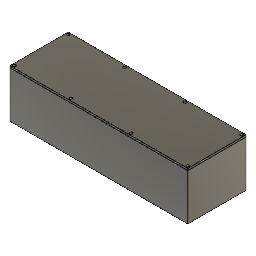
piPlayer (Autodesk Fusion 360 design; units mm, degrees)
Autodesk Fusion 360 part; units mm, degrees
note: some values were not read from the file. Set by a fixed rule: which sketch regions a step uses.
sketch "Sketch1" plane through (0, 0, 0) normal (0, 0, 1) x (1, 0, 0) in component "Box"
  line L0 (0, 26.5) -> (-38, 26.5)
  line L1 (-38, 26.5) -> (-38, -26.5)
  line L2 (-38, -26.5) -> (0, -26.5)
  line L3 (0, -26.5) -> (0, 26.5)
  line L4 (-38, -26.5) -> (-91, -26.5)
  line L5 (-91, -26.5) -> (-91, 26.5)
  line L6 (-91, 26.5) -> (-38, 26.5)
  line L7 (-91, 26.5) -> (-38, -26.5) construction
  line L8 (-38, 26.5) -> (-91, -26.5) construction
  circle A0 centre (-64.5, 0) radius 26.5
  circle A1 centre (-85.7132, 21.2132) radius 2
  circle A2 centre (-43.2868, 21.2132) radius 2
  circle A3 centre (-43.2868, -21.2132) radius 2
  circle A4 centre (-85.7132, -21.2132) radius 2
  line L9 (0, 31.5) -> (-96, 31.5)
  line L10 (-96, 31.5) -> (-96, -31.5)
  line L11 (-96, -31.5) -> (0, -31.5)
  line L12 (0, -31.5) -> (0, -26.5)
  line L13 (0, 31.5) -> (0, 26.5)
  line L14 (-36, -26.5) -> (-36, 26.5)
  circle A5 centre (-29, 0.4958) radius 4
  circle A6 centre (-29, 0.4958) radius 3
  circle A7 centre (-28.5622, -22.5) radius 1.5
  circle A8 centre (-28.5622, -22.5) radius 4
  dimension "d10" = 38
  dimension "d11" = 53
  dimension "d12" = 53
  dimension "d13" = 53
  dimension "d14" = 4
  dimension "d15" = 60
  dimension "d16" = 5
  dimension "d17" = 5
  dimension "d18" = 5
  dimension "d23" = 2
  dimension "d30" = 8
  dimension "d31" = 6
  dimension "d32" = 29
  dimension "d53" = 23
  dimension "d54" = 3
  dimension "d55" = 8
  constraint horizontal L0
  constraint vertical L1
  constraint horizontal L2
  constraint vertical L3
  constraint coincident origin L3
  constraint horizontal L4
  constraint vertical L5
  constraint horizontal L6
  constraint collinear L0 L6
  constraint midpoint L8 A0.centre
  constraint midpoint origin L3
  constraint coincident L7 A1.centre
  constraint coincident L8 A2.centre
  constraint coincident L7 A3.centre
  constraint coincident L8 A4.centre
  constraint equal A1 A2
  constraint equal A1 A3
  constraint equal A1 A4
  constraint horizontal A1.centre A2.centre
  constraint vertical A2.centre A3.centre
  constraint horizontal A3.centre A4.centre
  constraint perpendicular L3 L9
  constraint perpendicular L9 L10
  constraint perpendicular L3 L11
  constraint perpendicular L2 L12
  constraint perpendicular L0 L13
  constraint coincident L2 L14.start
  constraint coincident L0 L14.end
  constraint perpendicular L0 L14
  constraint concentric A5 A6
  constraint concentric A7 A8
  constraint tangent L2 A8
  measures "d10" distance of L0.start L0.end
  measures "d11" distance of L5.end L0.end
  measures "d12" distance of L4.end L5.end
  measures "d13" diameter of A0
  measures "d14" diameter of A1
  measures "d15" distance of A2.centre A4.centre
  measures "d16" distance of L0 L9
  measures "d17" distance of L5 L10
  measures "d18" distance of L4 L11
  measures "d23" distance of L1 L14
  measures "d30" diameter of A5
  measures "d31" diameter of A6
  measures "d32" distance of L3 A5.centre
  measures "d53" distance of A5.centre A7.centre
  measures "d54" diameter of A7
  measures "d55" diameter of A8
extrude "Extrude1" add sketch "Sketch1" along normal blind 2 contours A8 | L0 L2 L3 L14 | L0 L1 L2 L14 | L1 L6 A0 | L1 L4 A0 | L5 L6 A0 | L4 L5 A0 | A5 | A6 | A7 makes body 1 at (-12.6914, -0.6601, 0) in component "Box"
extrude "Extrude2" add sketch "Sketch1" along normal blind 50 contours L0 L2 L4 L5 L6 L9 L10 L11 L12 L13 | L0 L1 L2 L14 bodies 1 in component "Box"
sketch "Sketch2" plane through (-36, 0, 0) normal (1, 0, 0) x (0, 1, 0) in component "Box"
  line L0 (-26.5, 2) -> (26.5, 2)
  line L1 (26.5, 2) -> (26.5, 50)
  line L2 (26.5, 50) -> (-26.5, 50)
  line L3 (-26.5, 50) -> (-26.5, 2)
  circle A0 centre (19.3, 20) radius 1.1
  circle A1 centre (21.5, 20) radius 1.1
  line L4 (19.6899, 21.0286) -> (21.1101, 21.0286)
  line L5 (19.6848, 18.9695) -> (21.1152, 18.9695)
  line L6 (-31.5, 0) -> (31.5, 0)
  line L7 (31.5, 0) -> (31.5, 50)
  dimension "d24" = 2.2
  dimension "d56" = 2.2
  dimension "d64" = 20
  dimension "d65" = 10
  constraint horizontal A0.centre A1.centre
  constraint tangent A0 A1
  constraint coincident A0 L4.start
  constraint coincident A1 L4.end
  constraint horizontal L4
  constraint coincident A0 L5.start
  constraint coincident A1 L5.end
  constraint parallel L4 L5
  measures "d24" diameter of A0
  measures "d56" diameter of A1
  measures "d64" distance of A1.centre L6
  measures "d65" distance of A1.centre L7
extrude "Extrude3" cut sketch "Sketch2" against normal up to surface (2 mm away) contours A0 | A0 A1 L5 | A0 A1 L4 | A1 bodies 1 in component "Box"
extrude "Extrude4" add sketch "Sketch1" along normal blind 10 contours A8 | A5 bodies 1 in component "Box"
sketch "Sketch4" plane through (0, 0, 50) normal (0, 0, 1) x (-1, 0, 0) in component "Box"
  line L0 (91, 26.5) -> (91, -26.5)
  line L1 (91, -26.5) -> (38, -26.5)
  line L2 (38, -26.5) -> (38, 26.5)
  line L3 (38, 26.5) -> (91, 26.5)
  line L4 (0, -31.5) -> (96, -31.5)
  line L5 (96, -31.5) -> (96, 31.5)
  line L6 (96, 31.5) -> (0, 31.5)
  line L7 (0, 31.5) -> (0, 26.5)
  line L8 (0, 26.5) -> (36, 26.5)
  line L9 (36, 26.5) -> (36, -26.5)
  line L10 (36, -26.5) -> (0, -26.5)
  line L11 (0, -26.5) -> (0, -31.5)
  line L12 (91, -26.5) -> (96, -31.5) construction
  circle A0 centre (93.5, -29) radius 1.5
  line L13 (96, 0) -> (36, 0) construction
  circle A1 centre (93.5, 29) radius 1.5
  circle A2 centre (32.5, -29) radius 1.5
  circle A3 centre (32.5, 29) radius 1.5
  dimension "d43" = 3
  dimension "d50" = -61
  dimension "d51" = 0
  constraint coincident L0.end L1.start
  constraint coincident L4.end L5.start
  constraint midpoint L12 A0.centre
  constraint midpoint L5 L13.start
  constraint midpoint L9 L13.end
  constraint symmetric A0 L13 A1
  measures "d43" diameter of A0
extrude "Extrude5" cut sketch "Sketch4" against normal blind 20 contours A0 | A1 | A2 | A3 bodies 1 in component "Box"
sketch "Sketch1 (2)" plane through (0, 0, 50) normal (0, 0, 1) x (-1, 0, 0) in component "Lid"
  circle A0 centre (93.5, -29) radius 1.5
  circle A1 centre (93.5, 29) radius 1.5
  line L0 (91, 26.5) -> (91, -26.5)
  line L1 (91, -26.5) -> (38, -26.5)
  line L2 (38, -26.5) -> (38, 26.5)
  line L3 (38, 26.5) -> (91, 26.5)
  line L4 (0, -31.5) -> (96, -31.5)
  line L5 (96, -31.5) -> (96, 31.5)
  line L6 (96, 31.5) -> (0, 31.5)
  line L7 (36, 26.5) -> (36, -26.5)
  line L8 (96, -31.5) -> (0, -31.5)
  line L9 (0, -31.5) -> (0, 31.5)
  line L10 (0, 31.5) -> (96, 31.5)
  line L11 (96, 31.5) -> (96, -31.5)
  circle A2 centre (93.5, -29) radius 1.5
  circle A3 centre (93.5, 29) radius 1.5
  circle A4 centre (32.5, -29) radius 1.5
  circle A5 centre (32.5, 29) radius 1.5
  line L12 (0, 31.5) -> (0, 26.5)
  line L13 (0, 26.5) -> (36, 26.5)
  line L14 (36, -26.5) -> (0, -26.5)
  line L15 (0, -26.5) -> (0, -31.5)
  constraint horizontal L8
  constraint vertical L9
  constraint horizontal L10
  constraint vertical L11
  constraint coincident L6.end L9.end
  constraint coincident L4.end L5.start
extrude "Extrude1'" add sketch "Sketch1 (2)" along normal blind 2 separate body contours L0 L1 L2 L3 | L4 L5 L6 L7 L8 L9 L10 L11 L12 L13 L14 L15 | L7 L9 L13 L14 makes body 2 in component "Lid"
mirror "Mirror1" about plane through (0, -31.5, 0) normal (1, 0, 0) of bodies 1 makes body 3 in component "Box"
combine "Combine1" operation add target body 1 tool bodies 3 in component "Box"
mirror "Mirror1'" about plane through (0, 31.5, 50) normal (1, 0, 0) of bodies 2 makes body 4 in component "Lid"
combine "Combine1'" operation add target body 2 tool bodies 4 in component "Lid"
sketch "Sketch5" plane through (0, 31.5, 0) normal (0, 1, 0) x (-1, 0, 0) in component "Box"
  line L0 (-96, 0) -> (96, 0)
  line L1 (96, 0) -> (96, 50)
  line L2 (96, 50) -> (-96, 50)
  line L3 (-96, 50) -> (-96, 0)
  line L4 (-25, 2) -> (-33, 2)
  line L5 (25, 2) -> (33, 2)
  line L6 (36, 2) -> (28.5622, 2)
  line L7 (24.5622, 2) -> (32.5622, 2)
  line L8 (-24.5622, 2) -> (-32.5622, 2)
  line L9 (-28.5622, 2) -> (-36, 2)
  line L10 (-36, 2) -> (36, 2)
  line L11 (-36, 18.9) -> (-36, 21.1)
  line L12 (-36, 18.9) -> (-36, 21.1)
  line L13 (-36, 2) -> (-36, 50)
  line L14 (-36, 50) -> (-36, 2)
  line L15 (36, 18.9) -> (36, 21.1)
  line L16 (36, 18.9) -> (36, 21.1)
  line L17 (36, 2) -> (36, 50)
  line L18 (36, 50) -> (36, 2)
  line L19 (2.5, 8) -> (15.5, 8)
  line L20 (15.5, 8) -> (15.5, 15)
  line L21 (15.5, 15) -> (2.5, 15)
  line L22 (2.5, 15) -> (2.5, 8)
  line L23 (2.5, 11.5) -> (15.5, 11.5) construction
  line L24 (9, 15) -> (9, 8) construction
  line L25 (28.5622, 2) -> (-28.5622, 2)
  point P0 (-36, 21.0286)
  point P1 (-36, 18.9695)
  point P2 (36, 21.0286)
  point P3 (36, 18.9695)
  dimension "d58" = 13
  dimension "d59" = 7
  dimension "d60" = 9.5
  dimension "d61" = 27
  constraint horizontal L19
  constraint vertical L20
  constraint horizontal L21
  constraint vertical L22
  constraint midpoint L22 L23.start
  constraint midpoint L20 L23.end
  constraint midpoint L21 L24.start
  constraint midpoint L19 L24.end
  measures "d58" distance of L20.end L21.end
  measures "d59" distance of L19.end L20.end
  measures "d60" distance of L10 L23
  measures "d61" distance of L18 L24
extrude "Extrude6" cut sketch "Sketch5" against normal blind 5 contours L19 L20 L21 L22 bodies 1 in component "Box"
sketch "Sketch6" plane through (0, 0, 2) normal (0, 0, 1) x (-1, 0, 0) in component "Box"
  circle A0 centre (-29, -0.4958) radius 4
  circle A1 centre (29, -0.4958) radius 4
  line L0 (36, -26.5) -> (36, 26.5)
  line L1 (36, 26.5) -> (28.5622, 26.5)
  circle A2 centre (28.5622, 22.5) radius 4
  line L2 (28.5622, 26.5) -> (-28.5622, 26.5)
  circle A3 centre (-28.5622, 22.5) radius 4
  line L3 (-28.5622, 26.5) -> (-36, 26.5)
  line L4 (-36, 26.5) -> (-36, -26.5)
  line L5 (-36, -26.5) -> (36, -26.5)
  circle A4 centre (-14.5646, -15.4626) radius 3.65
  line L6 (-29, -0.4958) -> (-29, -26.5) construction
  line L7 (-29, -13.4979) -> (15.0999, -13.4979) construction
  dimension "d66" = 7.3
  constraint coincident A0.centre L6.start
  constraint coincident L5 L6.end
  constraint perpendicular L5 L6
  constraint midpoint L6 L7.start
  constraint perpendicular L6 L7
  measures "d66" diameter of A4
extrude "Extrude7" cut sketch "Sketch6" against normal up to surface (2 mm away) contours A4 bodies 1 in component "Box"
component "Box" placed x (1, 0, 0) y (0, 1, 0) z (0, 0, 1) at (0, 0, 0)
component "Lid" placed x (1, 0, 0) y (0, 1, 0) z (0, 0, 1) at (0, 0, 0)
equation "Pi_Width = 67 mm"
equation "Pi_Height = 30 mm"
equation "Speaker_Width = 53 mm"
equation "Speaker_Depth = 30 mm"
equation "Speaker_Mount_Spacing = 41 mm"
equation "Speaker_Mount_Diag = 60 mm"
equation "d10 = ( Pi_Width + 9 mm ) / 2"
equation "d11 = Speaker_Width"
equation "d12 = Speaker_Width"
equation "d15 = Speaker_Mount_Diag"
equation "d16 = Wall_Thickness"
equation "d17 = Wall_Thickness"
equation "d18 = Wall_Thickness"
equation "d21 = Speaker_Depth + 20 mm"
equation "d32 = ( Pi_Horiz_Hole_Dist / 2 )"
equation "Pi_Horiz_Hole_Dist = 58 mm"
equation "Pi_Vert_Hole_Dist = 23 mm"
equation "Wall_Thickness = 5 mm"
